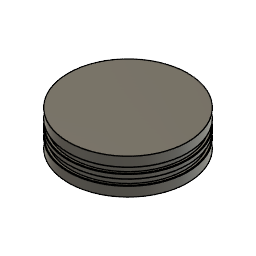
Piston head (Autodesk Fusion 360 design; units mm, degrees)
part number: 2026-04-29-16-39-42-460
Autodesk Fusion 360 part; units mm, degrees
sketch "Sketch1" plane through (0, 0, 0) normal (0, 1, 0) x (1, 0, 0)
  circle A0 centre (0, 0) radius 60
  dimension "d1" = 120
  constraint coincident A0.centre origin
  measures "d1" diameter of A0
extrude "Extrude1" add sketch "Sketch1" along normal blind 10
sketch "Sketch2" plane through (0, 10, 0) normal (0, 1, 0) x (-1, 0, 0)
  circle A0 centre (0, 0) radius 60
  circle A1 centre (0, 0) radius 57.4
  dimension "d4" = 114.8
  constraint coincident A0.centre A1.centre
  measures "d4" diameter of A1
extrude "Extrude2" add sketch "Sketch2" along normal blind 5.3 contours A1
sketch "Sketch3" plane through (0, 15.3, 0) normal (0, 1, 0) x (-1, 0, 0)
  circle A0 centre (0, 0) radius 57.4
  circle A1 centre (0, 0) radius 60
  dimension "d7" = 120
  constraint coincident A0.centre A1.centre
  measures "d7" diameter of A1
extrude "Extrude3" add sketch "Sketch3" along normal blind 5 contours A0 | A1
sketch "Sketch4" plane through (0, 20.3, 0) normal (0, 1, 0) x (-1, 0, 0)
  circle A0 centre (0, 0) radius 60
  circle A1 centre (0, 0) radius 57.4
  dimension "d10" = 114.8
  constraint coincident A0.centre A1.centre
  measures "d10" diameter of A1
extrude "Extrude4" add sketch "Sketch4" along normal blind 5.3 contours A1
sketch "Sketch5" plane through (0, 25.6, 0) normal (0, 1, 0) x (-1, 0, 0)
  circle A0 centre (0, 0) radius 57.4
  circle A1 centre (0, 0) radius 60
  dimension "d13" = 120
  constraint coincident A0.centre A1.centre
  measures "d13" diameter of A1
extrude "Extrude5" add sketch "Sketch5" along normal blind 10 contours A0 | A1
sketch "Sketch7" plane through (0, 0, 0) normal (0, -1, 0) x (1, 0, 0)
  circle A0 centre (0, 0) radius 60
  circle A1 centre (0, 0) radius 30
  dimension "d22" = 60
  constraint concentric A0 A1
  measures "d22" diameter of A1
extrude "Extrude7" cut sketch "Sketch7" against normal blind 10 contours A1
chamfer "Chamfer1" distance 0.5 angle 45 1 edges at (55.9396, 20.3, -21.6969)
chamfer "Chamfer2" distance 0.5 angle 45 3 edges at (55.9396, 25.6, -21.6969) (55.9396, 15.3, -21.6969) (-55.9396, 10, 21.6969)
